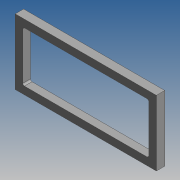
# Autodesk Inventor part: P031_MonoVitreBas
Saved by Autodesk Inventor 2021.3 (Build 253353000, 353)
## iProperties
Created: 2021-11-12
Part Number: P031_MonoVitreBas
Material: Générique
Document SubType Name: Modeling
Designer: gabri
Density: 1 g/cm^3
Appearance: Par défaut
Author: gabri
Autodesk Inventor part; units mm, degrees
ref_plane "YZ Plane" through (0, 0, 0) normal (1, 0, 0) x (0, 1, 0)
ref_plane "XZ Plane" through (0, 0, 0) normal (0, 1, 0) x (-1, 0, 0)
ref_plane "XY Plane" through (0, 0, 0) normal (0, 0, 1) x (1, 0, 0)
sketch "Sketch2" plane through (0, 0, 0) normal (0, 1, 0) x (-1, 0, 0)
  line L0 (-75, -30) -> (75, -30)
  line L1 (75, -30) -> (75, 30)
  line L2 (75, 30) -> (-75, 30)
  line L3 (-75, 30) -> (-75, -30)
  line L4 (-75, -30) -> (75, 30) construction
  line L5 (75, -30) -> (-75, 30) construction
  line L6 (-84, -39) -> (84, -39)
  line L7 (84, -39) -> (84, 39)
  line L8 (84, 39) -> (-84, 39)
  line L9 (-84, 39) -> (-84, -39)
  line L10 (-84, -39) -> (84, 39) construction
  line L11 (84, -39) -> (-84, 39) construction
  point P0 (0, 0)
  dimension "d0" = 150
  dimension "d1" = 60
  dimension "d4" = 9
  dimension "d5" = 9
  dimension "d53" = 168
  dimension "d54" = 78
  constraints: 24 end point, 4 midpoint, 4 parallel, 2 horizontal, 2 perpendicular
  measures "d0" distance of L1.end L2.end
  measures "d1" distance of L0.end L1.end
  measures "d4" distance between parallel lines of L8 L2
  measures "d5" distance between parallel lines of L1 L7
  measures "d53" distance of L6.start L6.end
  measures "d54" distance of L8.end L6.start
extrude "Extrusion1" add sketch "Sketch2" along normal blind 10
sketch "Sketch4" plane through (0, 10, 0) normal (0, 1, 0) x (1, 0, 0)
  line L0 (-84, 39) -> (-84, -39) construction
  line L1 (-84, -39) -> (84, -39) construction
  line L2 (84, -39) -> (84, 39) construction
  line L3 (84, 39) -> (-84, 39) construction
  line L4 (75, 30) -> (75, -30) construction
  line L5 (75, -30) -> (-75, -30) construction
  line L6 (-75, -30) -> (-75, 30) construction
  line L7 (-75, 30) -> (75, 30) construction
  line L8 (-75, 30) -> (75, 30)
  line L9 (75, 30) -> (75, -30)
  line L10 (75, -30) -> (-75, -30)
  line L11 (-75, -30) -> (-75, 30)
  line L12 (-75, 30) -> (75, -30) construction
  line L13 (75, 30) -> (-75, -30) construction
  line L14 (-79, 34) -> (79, 34)
  line L15 (79, 34) -> (79, -34)
  line L16 (79, -34) -> (-79, -34)
  line L17 (-79, -34) -> (-79, 34)
  line L18 (-79, 34) -> (79, -34) construction
  line L19 (79, 34) -> (-79, -34) construction
  point P0 (0, 0)
  dimension "d8" = 4
  dimension "d9" = 4
  constraints: 24 end point, 4 midpoint, 4 parallel, 2 horizontal, 2 perpendicular
  measures "d8" distance between parallel lines of L16 L10
  measures "d9" distance between parallel lines of L4 L15
extrude "Extrusion2" cut sketch "Sketch4" against normal blind 1
sketch "Sketch7" plane through (0, 9, 0) normal (0, 1, 0) x (1, 0, 0)
  line L0 (79, -34) -> (-79, -34) construction
  line L1 (79, 34) -> (79, -34) construction
  line L2 (-79, 34) -> (79, 34) construction
  line L3 (-79, -34) -> (-79, 34) construction
  line L4 (75, 30) -> (-75, 30) construction
  line L5 (75, -30) -> (75, 30) construction
  line L6 (-75, -30) -> (75, -30) construction
  line L7 (-75, 30) -> (-75, -30) construction
  line L8 (-76, 31) -> (76, 31)
  line L9 (76, 31) -> (76, -31)
  line L10 (76, -31) -> (-76, -31)
  line L11 (-76, -31) -> (-76, 31)
  line L12 (-76, 31) -> (76, -31) construction
  line L13 (76, 31) -> (-76, -31) construction
  line L14 (-79, 34) -> (79, 34)
  line L15 (79, 34) -> (79, -34)
  line L16 (79, -34) -> (-79, -34)
  line L17 (-79, -34) -> (-79, 34)
  line L18 (-79, 34) -> (79, -34) construction
  line L19 (79, 34) -> (-79, -34) construction
  point P0 (0, 0)
  dimension "d15" = 3
  dimension "d16" = 3
  constraints: 24 end point, 4 midpoint, 4 parallel, 2 horizontal, 2 perpendicular
  measures "d15" distance between parallel lines of L10 L0
  measures "d16" distance between parallel lines of L9 L15
extrude "Extrusion3" cut sketch "Sketch7" against normal blind 2.5
fillet "Fillet1" radius 2 8 edges at (76, 7.75, 31) (-76, 7.75, 31) (-76, 7.75, -31) (76, 7.75, -31) (75, 4.5, 30) (75, 4.5, -30) (-75, 4.5, -30) (-75, 4.5, 30)
fillet "Fillet2" radius 2 4 edges at (79, 8.25, 34) (79, 8.25, -34) (-79, 8.25, 34) (-79, 8.25, -34)
sketch "Sketch8" plane through (0, 10, 0) normal (0, 1, 0) x (1, 0, 0)
  line L0 (79, 32) -> (79, -32) construction
  arc A0 (77, -34) -> (79, -32) centre (77, -32) ccw construction
  line L1 (77, -34) -> (-77, -34) construction
  arc A1 (-79, -32) -> (-77, -34) centre (-77, -32) ccw construction
  line L2 (-79, -32) -> (-79, 32) construction
  arc A2 (-77, 34) -> (-79, 32) centre (-77, 32) ccw construction
  line L3 (-77, 34) -> (77, 34) construction
  arc A3 (79, 32) -> (77, 34) centre (77, 32) ccw construction
  line L4 (-84, 39) -> (-84, -39) construction
  line L5 (-84, -39) -> (84, -39) construction
  line L6 (84, -39) -> (84, 39) construction
  line L7 (84, 39) -> (-84, 39) construction
  line L8 (152.6, 0) -> (-152.6, 0) construction
  line L9 (0, 68.6) -> (0, -68.6) construction
  line L10 (-75, 28) -> (-75, -28) construction
  line L11 (73, 30) -> (-73, 30) construction
  line L12 (75, -28) -> (75, 28) construction
  line L13 (-73, -30) -> (73, -30) construction
  point P0 (0, 0)
  point P1 (81, -36)
  point P2 (81, 0)
  point P3 (81, 36)
  point P4 (0, 36)
  point P5 (-81, 36)
  point P6 (-81, 0)
  point P7 (-81, -36)
  point P8 (0, -36)
  dimension "d21" = 5
  dimension "d41" = 6
  dimension "d42" = 6
  dimension "d43" = 6
  dimension "d44" = 6
  dimension "d45" = 6
  dimension "d46" = 6
  dimension "d47" = 6
  dimension "d48" = 6
  dimension "d49" = 6
  dimension "d50" = 6
  dimension "d51" = 6
  dimension "d52" = 6
  constraints: 4 point on line
  measures "d21" distance between parallel lines of L7 L3
  measures "d41" distance from line of L10 point (-81, 36)
  measures "d42" distance from line of L11 point (-81, 36)
  measures "d43" distance from line of L11 point (0, 36)
  measures "d44" distance from line of L11 point (81, 36)
  measures "d45" distance from line of L12 point (81, 36)
  measures "d46" distance from line of L12 point (81, 0)
  measures "d47" distance from line of L13 point (81, -36)
  measures "d48" distance from line of L12 point (81, -36)
  measures "d49" distance from line of L13 point (0, -36)
  measures "d50" distance from line of L13 point (-81, -36)
  measures "d51" distance from line of L10 point (-81, -36)
  measures "d52" distance from line of L10 point (-81, 0)
hole "Hole1" at (81, 10, 36) at (81, 10, 0) at (81, 10, -36) at (0, 10, -36) at (-81, 10, -36) at (-81, 10, 0) at (-81, 10, 36) at (0, 10, 36) direction (0, -1, 0) diameter 2.459 depth 8.8 tip angle 118 thread size "M3x0.5" class "6H" standard "ISO Metric profile"
body "Solid1"
